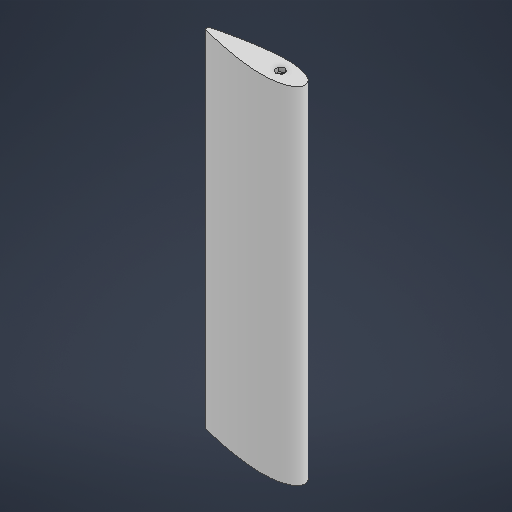
# Autodesk Inventor part: Elevon
Saved by Autodesk Inventor 2026 (Build 300175050, 175E)
## iProperties
Created: 2026-07-28
Part Number: Elevon
Material: Generic
Document SubType Name: Modeling
Designer: Delbe
Density: 1 g/cm^3
Appearance: Default
Author: Delbe
Autodesk Inventor part; units mm, degrees
ref_plane "YZ Plane" through (0, 0, 0) normal (1, 0, 0) x (0, 1, 0)
ref_plane "XZ Plane" through (0, 0, 0) normal (0, 1, 0) x (-1, 0, 0)
ref_plane "XY Plane" through (0, 0, 0) normal (0, 0, 1) x (1, 0, 0)
sketch "Sketch1" plane through (0, 0, 0) normal (0, 1, 0) x (-1, 0, 0)
  spline S0 degree 4 poles (88.62, 0.2278) (88.5883, 0.2369) (88.4338, 0.281) (88.1748, 0.355) (87.7378, 0.4789) (87.2791, 0.6082) (86.717, 0.7656) (86.0569, 0.9489) (85.2986, 1.1575) (84.4448, 1.3897) (83.4971, 1.6444) (82.4578, 1.92) (81.3295, 2.2149) (80.1146, 2.5276) (78.8162, 2.8562) (77.4371, 3.1993) (75.9807, 3.5549) (74.4502, 3.9213) (72.8494, 4.2967) (71.182, 4.6793) (69.4517, 5.0673) (67.6628, 5.4589) (65.8193, 5.8521) (63.9255, 6.2451) (61.986, 6.6359) (60.0052, 7.0225) (57.9877, 7.403) (55.9383, 7.7751) (53.8617, 8.1368) (51.7629, 8.4859) (49.6466, 8.8201) (47.5178, 9.1371) (45.3815, 9.4346) (43.2427, 9.7103) (41.1064, 9.9618) (38.9775, 10.1867) (36.861, 10.3829) (34.7619, 10.548) (32.6849, 10.68) (30.6351, 10.777) (28.6171, 10.837) (26.6357, 10.8585) (24.6954, 10.8401) (22.8009, 10.7806) (20.9564, 10.6792) (19.1664, 10.5352) (17.4349, 10.3484) (15.766, 10.1187) (14.1636, 9.8465) (12.6314, 9.5325) (11.1729, 9.1773) (9.7915, 8.7824) (8.4905, 8.3489) (7.2726, 7.8786) (6.1408, 7.3731) (5.0975, 6.8344) (4.1451, 6.2642) (3.2858, 5.6644) (2.5214, 5.0367) (1.8539, 4.383) (1.2849, 3.7045) (0.8162, 3.0027) (0.4497, 2.2791) (0.1872, 1.5351) (0.03, 0.7753) (-0.0214, 0) (0.03, -0.7753) (0.1872, -1.5351) (0.4497, -2.2791) (0.8162, -3.0027) (1.2849, -3.7045) (1.8539, -4.383) (2.5214, -5.0367) (3.2858, -5.6644) (4.1451, -6.2642) (5.0975, -6.8344) (6.1408, -7.3731) (7.2726, -7.8786) (8.4905, -8.3489) (9.7915, -8.7824) (11.1729, -9.1773) (12.6314, -9.5325) (14.1636, -9.8465) (15.766, -10.1187) (17.4349, -10.3484) (19.1664, -10.5352) (20.9564, -10.6792) (22.8009, -10.7806) (24.6954, -10.8401) (26.6357, -10.8585) (28.6171, -10.837) (30.6351, -10.777) (32.6849, -10.68) (34.7619, -10.548) (36.861, -10.3829) (38.9775, -10.1867) (41.1064, -9.9618) (43.2427, -9.7103) (45.3815, -9.4346) (47.5178, -9.1371) (49.6466, -8.8201) (51.7629, -8.4859) (53.8617, -8.1368) (55.9383, -7.7751) (57.9877, -7.403) (60.0052, -7.0225) (61.986, -6.6359) (63.9255, -6.2451) (65.8193, -5.8521) (67.6628, -5.4589) (69.4517, -5.0673) (71.182, -4.6793) (72.8494, -4.2967) (74.4502, -3.9213) (75.9807, -3.5549) (77.4371, -3.1993) (78.8162, -2.8562) (80.1146, -2.5276) (81.3295, -2.2149) (82.4578, -1.92) (83.4971, -1.6444) (84.4448, -1.3897) (85.2986, -1.1575) (86.0569, -0.9489) (86.717, -0.7656) (87.2791, -0.6082) (87.7378, -0.4789) (88.1748, -0.355) (88.4338, -0.281) (88.5883, -0.2369) (88.62, -0.2278) knots 0 0 0 0 0 0.00622 0.009879 0.014135 0.018903 0.024123 0.029751 0.035753 0.042099 0.048763 0.055721 0.062954 0.070443 0.078169 0.086116 0.094269 0.102613 0.111133 0.119816 0.128647 0.137615 0.146707 0.155909 0.16521 0.174597 0.184059 0.193583 0.203159 0.212773 0.222415 0.232073 0.241736 0.251392 0.261031 0.27064 0.28021 0.28973 0.299188 0.308575 0.31788 0.327093 0.336204 0.345204 0.354082 0.362831 0.37144 0.379902 0.388209 0.396351 0.404321 0.412114 0.419721 0.427138 0.43436 0.441385 0.448212 0.454844 0.461288 0.467554 0.473662 0.479636 0.485511 0.491326 0.497112 0.502888 0.508674 0.514489 0.520364 0.526338 0.532446 0.538712 0.545156 0.551788 0.558615 0.56564 0.572862 0.580279 0.587886 0.595679 0.603649 0.611791 0.620098 0.62856 0.637169 0.645918 0.654796 0.663796 0.672907 0.68212 0.691425 0.700812 0.71027 0.71979 0.72936 0.738969 0.748608 0.758264 0.767927 0.777585 0.787227 0.796841 0.806417 0.815941 0.825403 0.83479 0.844091 0.853293 0.862385 0.871353 0.880184 0.888867 0.897387 0.905731 0.913884 0.921831 0.929557 0.937046 0.944279 0.951237 0.957901 0.964247 0.970249 0.975877 0.981097 0.985865 0.990121 0.99378 1 1 1 1 1
  line L0 (88.62, 0.2278) -> (88.62, -0.2278)
  line L1 (88.4131, 0.2869) -> (88.4131, -0.2869)
  line L2 (88.4131, 0) -> (85.4131, 0) construction
  line L3 (85.3488, -1.1432) -> (85.3488, 1.1432)
  line L4 (85.3488, 0) -> (84.3488, 0) construction
  line L5 (84.3488, -1.415) -> (84.3488, 1.415)
  line L6 (84.3488, 0) -> (82.3488, 0) construction
  line L7 (82.3488, 0) -> (82.3488, -1.9478)
  line L8 (82.3488, 0) -> (82.3488, 1.9478)
  point P0 (0, 0)
  point P1 (88.5683, 0.2426)
  point P2 (88.155, 0.3604)
  point P3 (87.7945, 0.4627)
  point P4 (87.3324, 0.593)
  point P5 (86.7699, 0.7506)
  point P6 (86.1081, 0.9344)
  point P7 (84.4936, 1.3759)
  point P8 (83.5446, 1.631)
  point P9 (82.5039, 1.907)
  point P10 (81.374, 2.2024)
  point P11 (80.1575, 2.5155)
  point P12 (78.8574, 2.8447)
  point P13 (77.4765, 3.1882)
  point P14 (76.0182, 3.5443)
  point P15 (74.4858, 3.9112)
  point P16 (72.883, 4.2872)
  point P17 (71.2134, 4.6703)
  point P18 (69.481, 5.0589)
  point P19 (67.6897, 5.4509)
  point P20 (65.8439, 5.8447)
  point P21 (63.9478, 6.2381)
  point P22 (62.0058, 6.6294)
  point P23 (60.0225, 7.0164)
  point P24 (58.0025, 7.3972)
  point P25 (55.9506, 7.7697)
  point P26 (53.8714, 8.1317)
  point P27 (51.7699, 8.481)
  point P28 (49.651, 8.8154)
  point P29 (47.5196, 9.1325)
  point P30 (45.3807, 9.4301)
  point P31 (43.2393, 9.7057)
  point P32 (41.1004, 9.9571)
  point P33 (38.969, 10.1818)
  point P34 (36.8501, 10.3776)
  point P35 (34.7486, 10.5424)
  point P36 (32.6694, 10.6739)
  point P37 (30.6175, 10.7702)
  point P38 (28.5975, 10.8295)
  point P39 (26.6142, 10.8502)
  point P40 (24.6722, 10.8309)
  point P41 (22.7761, 10.7703)
  point P42 (20.9303, 10.6678)
  point P43 (19.139, 10.5225)
  point P44 (17.4066, 10.3344)
  point P45 (15.737, 10.1033)
  point P46 (14.1342, 9.8295)
  point P47 (12.6018, 9.5138)
  point P48 (11.1435, 9.157)
  point P49 (9.7626, 8.7602)
  point P50 (8.4625, 8.3249)
  point P51 (7.246, 7.8528)
  point P52 (6.1161, 7.3455)
  point P53 (5.0754, 6.805)
  point P54 (4.1264, 6.2333)
  point P55 (3.2712, 5.6325)
  point P56 (2.5119, 5.0046)
  point P57 (1.8501, 4.3516)
  point P58 (1.2876, 3.6754)
  point P59 (0.8255, 2.9776)
  point P60 (0.465, 2.26)
  point P61 (0.2069, 1.5238)
  point P62 (0.0517, 0.7702)
  point P63 (0, 0)
  point P64 (0.0517, -0.7702)
  point P65 (0.2069, -1.5238)
  point P66 (0.465, -2.26)
  point P67 (0.8255, -2.9776)
  point P68 (1.2876, -3.6754)
  point P69 (1.8501, -4.3516)
  point P70 (2.5119, -5.0046)
  point P71 (3.2712, -5.6325)
  point P72 (4.1264, -6.2333)
  point P73 (5.0754, -6.805)
  point P74 (6.1161, -7.3455)
  point P75 (7.246, -7.8528)
  point P76 (8.4625, -8.3249)
  point P77 (9.7626, -8.7602)
  point P78 (11.1435, -9.157)
  point P79 (12.6018, -9.5138)
  point P80 (14.1342, -9.8295)
  point P81 (15.737, -10.1033)
  point P82 (17.4066, -10.3344)
  point P83 (19.139, -10.5225)
  point P84 (20.9303, -10.6678)
  point P85 (22.7761, -10.7703)
  point P86 (24.6722, -10.8309)
  point P87 (26.6142, -10.8502)
  point P88 (28.5975, -10.8295)
  point P89 (30.6175, -10.7702)
  point P90 (32.6694, -10.6739)
  point P91 (34.7486, -10.5424)
  point P92 (36.8501, -10.3776)
  point P93 (38.969, -10.1818)
  point P94 (41.1004, -9.9571)
  point P95 (43.2393, -9.7057)
  point P96 (45.3807, -9.4301)
  point P97 (47.5196, -9.1325)
  point P98 (49.651, -8.8154)
  point P99 (51.7699, -8.481)
  point P100 (53.8714, -8.1317)
  point P101 (55.9506, -7.7697)
  point P102 (58.0025, -7.3972)
  point P103 (60.0225, -7.0164)
  point P104 (62.0058, -6.6294)
  point P105 (63.9478, -6.2381)
  point P106 (65.8439, -5.8447)
  point P107 (67.6897, -5.4509)
  point P108 (69.481, -5.0589)
  point P109 (71.2134, -4.6703)
  point P110 (72.883, -4.2872)
  point P111 (74.4858, -3.9112)
  point P112 (76.0182, -3.5443)
  point P113 (77.4765, -3.1882)
  point P114 (78.8574, -2.8447)
  point P115 (80.1575, -2.5155)
  point P116 (81.374, -2.2024)
  point P117 (82.5039, -1.907)
  point P118 (83.5446, -1.631)
  point P119 (84.4936, -1.3759)
  point P120 (85.3488, -1.1432)
  point P121 (86.1081, -0.9344)
  point P122 (86.7699, -0.7506)
  point P123 (87.3324, -0.593)
  point P124 (87.7945, -0.4627)
  point P125 (88.155, -0.3604)
  point P126 (88.5683, -0.2426)
  dimension "d33" = 3
  dimension "d45" = 1
  dimension "d52" = 2
  constraints: 18 end point, 4 vertical, 3 horizontal, 2 midpoint, 1 perpendicular, 1 point on line, 136 other
  measures "d33" distance of L2.start L2.end
  measures "d45" distance of L4.start L4.end
  measures "d52" distance of L4.end L6.end
extrude "Extrusion1" add sketch "Sketch1" along normal blind 296 contours L5 S0 L7 L8 | L8 L7 S0
sketch "Sketch2" plane through (0, 296, 0) normal (0, 1, 0) x (1, 0, 0)
  line L0 (2, 0) -> (-21.125, 0) construction
  circle A0 centre (-21.125, 0) radius 1.75 construction
  line L1 (-21.125, 0) -> (-21.125, 2) construction
  point P0 (0, 0)
  dimension "d2" = 21.125
  dimension "d3" = 3.5
  dimension "d46" = 2
  constraints: 4 end point, 1 centre point, 1 coincident, 1 horizontal, 1 vertical
  measures "d2" distance of point (0, 0) L0.end
  measures "d3" diameter of A0
  measures "d46" distance of L1.start L1.end
hole "Hole1" at (-21.125, 296, 0) direction (0, -1, 0) diameter 4.5 end through all
sketch "Sketch3" plane through (0, 296, 0) normal (0, 1, 0) x (1, 0, 0)
  line L0 (2, 0) -> (-21.125, 0)
  line L1 (-26.6253, 0.5) -> (-23.6253, 0.5) construction
  line L2 (-17.625, 0) -> (-24.625, 0) construction
  line L3 (-21.125, 0) -> (-21.125, 2) construction
  line L4 (-0.0003, -2) -> (-0.0003, 0) construction
  line L5 (-17.625, 2) -> (-17.625, -2)
  line L6 (-24.625, 2) -> (-24.625, -2)
  line L7 (-24.625, 2) -> (-21.1609, 4)
  line L8 (-24.625, 2) -> (-20.625, 2) construction
  line L9 (-21.1609, 4) -> (-17.625, 2)
  line L10 (-24.625, -2) -> (-21.1609, -4)
  line L11 (-21.1609, -4) -> (-17.625, -2)
  point P0 (0, 0)
  dimension "d11" = 21.125
  dimension "d18" = 7
  dimension "d56" = 4
  constraints: 24 end point, 4 horizontal, 3 midpoint, 2 vertical, 1 equal length, 1 parallel
  measures "d11" distance of point (0, 0) L0.end
  measures "d18" distance of L2.start L2.end
  measures "d56" distance of L6.start L7.end
extrude "Extrusion2" cut sketch "Sketch3" against normal blind 3.5
sketch "Sketch4" plane through (0, 0, 0) normal (0, -1, 0) x (1, 0, 0)
  line L0 (1.9997, 0) -> (-21.125, 0) construction
  circle A0 centre (-21.125, 0) radius 4.25
  line L1 (-21.125, 0) -> (-45.625, 0)
  line L2 (-21.125, 0) -> (-16.625, 0)
  line L3 (-45.625, 2.75) -> (-45.625, -2.75)
  line L4 (-45.625, 2.75) -> (-21.1246, 4.25)
  line L5 (-45.625, -2.75) -> (-21.1254, -4.25)
  line L6 (-16.625, 0) -> (-16.625, 4.5255)
  line L7 (-16.625, 4.5255) -> (-21.1246, 4.25)
  line L8 (-21.1254, -4.25) -> (-16.625, -4.5255)
  line L9 (-16.625, 0) -> (-16.625, -4.5255)
  circle A1 centre (-21.125, 0) radius 4.5
  line L10 (-21.125, -4.5) -> (-45.625, -2.75)
  line L11 (-21.125, 4.5) -> (-45.625, 2.75)
  point P0 (0, 0)
  point P1 (-21.6431, -4.2183)
  point P2 (-21.6438, 4.2182)
  point P3 (-21.7646, 4.4543)
  point P4 (-21.7646, -4.4543)
  dimension "d24" = 21.125
  dimension "d25" = 8.5
  dimension "d26" = 24.5
  dimension "d27" = 4.5
  dimension "d28" = 5.5
  dimension "d31" = 9
  constraints: 24 end point, 4 point on circle, 4 point on line, 2 centre point, 2 coincident, 2 collinear, 2 horizontal, 2 vertical, 1 midpoint
  measures "d24" distance of point (0, 0) L0.end
  measures "d25" diameter of A0
  measures "d26" distance of L1.start L1.end
  measures "d27" distance of L1.start L2.end
  measures "d28" distance of L3.start L3.end
  measures "d31" diameter of A1
extrude "Extrusion3" cut sketch "Sketch4" against normal blind 3 contours L2 L1 A0 L4 | L2 A1 L8 A0 | A0 L5 L1 L2 | A0 L7 A1 L2 | L4 A0 | A0 L4 A1 L11 L7 | L8 A1 L10 L5 A0 | A0 L5 | A0 L1 A1 L4 | L5 A1 L1 A0 | A1 L1 L3 L4 | L4 L11 A1 | L11 A1 | A1 L10 L5 | L5 L3 L1 A1 | A1 L10
fillet "Fillet1" radius 2.5 2 edges at (-45.625, 1.5, -2.75) (-45.625, 1.5, 2.75)
sketch "Sketch5" plane through (0, 3, 0) normal (0, -1, 0) x (1, 0, 0)
  line L0 (-47.623, 0) -> (-41, 0) construction
  line L1 (-41, 0) -> (-40, 0) construction
  circle A0 centre (-40, 0) radius 1
  line L2 (-37.75, 0) -> (-36.75, 0) construction
  circle A1 centre (-36.75, 0) radius 1
  line L3 (-34.5, 0) -> (-33.5, 0) construction
  circle A2 centre (-33.5, 0) radius 1
  line L4 (-31.25, 0) -> (-30.25, 0) construction
  circle A3 centre (-30.25, 0) radius 1
  line L5 (-47.623, 0) -> (-47.623, 0) construction
  line L6 (-41, 0) -> (-39, 0)
  point P0 (0, 0)
  dimension "d34" = 6.623
  dimension "d35" = 1
  dimension "d38" = 3.25
  dimension "d50" = 0
  dimension "d51" = 2
  constraints: 14 end point, 4 coincident, 4 horizontal, 3 horizontal alignment, 2 point on circle, 1 centre point, 1 collinear, 1 line through centre, 1 point on line, 1 vertical, 17 other
  measures "d34" distance of L0.start L0.end
  measures "d35" distance of L0.end L1.end
  measures "d38" distance of L0.end L2.start
  measures "d50" distance of L0.start L5.end
  measures "d51" distance of L0.end L6.end
extrude "Extrusion4" cut sketch "Sketch5" against normal blind 5
body "Solid1"
